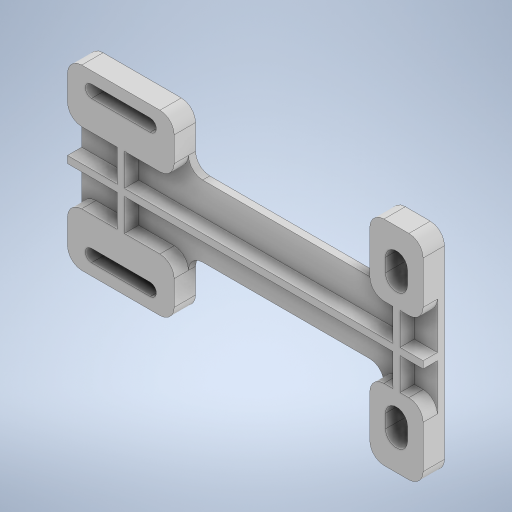
# Autodesk Inventor part: panel_holder
Saved by Autodesk Inventor 2023 (Build 270158000, 158)
## iProperties
Created: 2023-10-19
Part Number: panel_holder
Material: Generic
Document SubType Name: Modeling
Designer: mark
Density: 1 g/cm^3
Appearance: Default
Author: mark
Autodesk Inventor part; units mm, degrees
ref_plane "YZ Plane" through (0, 0, 0) normal (1, 0, 0) x (0, 1, 0)
ref_plane "XZ Plane" through (0, 0, 0) normal (0, 1, 0) x (-1, 0, 0)
ref_plane "XY Plane" through (0, 0, 0) normal (0, 0, 1) x (1, 0, 0)
sketch "Sketch1" plane through (0, 0, 0) normal (0, 0, 1) x (1, 0, 0)
  line L0 (0, 0) -> (-100, 0)
  line L1 (-100, 0) -> (-100, 50)
  line L2 (-100, 50) -> (0, 50)
  line L3 (0, 50) -> (0, 0)
  line L4 (-93.25, 46.75) -> (-76.75, 46.75)
  line L5 (-75, 45) -> (-75, 45)
  line L6 (-76.75, 43.25) -> (-93.25, 43.25)
  line L7 (-95, 45) -> (-95, 45)
  line L8 (-93.25, 6.75) -> (-76.75, 6.75)
  line L9 (-75, 5) -> (-75, 5)
  line L10 (-76.75, 3.25) -> (-93.25, 3.25)
  line L11 (-95, 5) -> (-95, 5)
  arc A0 (-93.25, 46.75) -> (-95, 45) centre (-93.25, 45) ccw
  arc A1 (-95, 45) -> (-93.25, 43.25) centre (-93.25, 45) ccw
  arc A2 (-75, 45) -> (-76.75, 46.75) centre (-76.75, 45) ccw
  arc A3 (-76.75, 43.25) -> (-75, 45) centre (-76.75, 45) ccw
  arc A4 (-75, 5) -> (-76.75, 6.75) centre (-76.75, 5) ccw
  arc A5 (-93.25, 6.75) -> (-95, 5) centre (-93.25, 5) ccw
  arc A6 (-95, 5) -> (-93.25, 3.25) centre (-93.25, 5) ccw
  arc A7 (-76.75, 3.25) -> (-75, 5) centre (-76.75, 5) ccw
  line L12 (0, 55) -> (-15, 55)
  line L13 (-15, 55) -> (-15, -5)
  line L14 (-15, -5) -> (0, -5)
  line L15 (0, -5) -> (0, 55)
  line L16 (-70, 50) -> (-15, 50)
  line L17 (-15, 50) -> (-15, 35)
  line L18 (-15, 35) -> (-70, 35)
  line L19 (-70, 35) -> (-70, 50)
  line L20 (-70, 0) -> (-15, 0)
  line L21 (-15, 0) -> (-15, 15)
  line L22 (-15, 15) -> (-70, 15)
  line L23 (-70, 15) -> (-70, 0)
  point P0 (-75, 43.25)
  point P1 (-75, 46.75)
  point P2 (-95, 43.25)
  point P3 (-95, 6.75)
  point P4 (-75, 3.25)
  point P5 (-75, 6.75)
  dimension "d0" = 100
  dimension "d1" = 50
  dimension "d2" = 20
  dimension "d3" = 3.5
  dimension "d4" = 3.5
  dimension "d5" = 36.5
  dimension "d6" = 3.25
  dimension "d7" = 5
  dimension "d8" = 1.75
  dimension "d11" = 15
  dimension "d12" = 60
  dimension "d13" = 15
  dimension "d14" = 15
  dimension "d17" = 55
  dimension "d18" = 15
  dimension "d19" = 5
  constraints: 48 end point, 19 point on line, 16 point on circle, 16 tangent, 12 parallel, 8 centre point, 7 equal radius, 6 horizontal, 6 perpendicular, 1 midpoint
  measures "d0" distance of L1.end L2.end
  measures "d1" distance of L0.end L1.end
  measures "d2" distance of point (-75, 43.25) point (-95, 43.25)
  measures "d3" distance of point (-75, 46.75) point (-75, 43.25)
  measures "d4" distance of point (-75, 6.75) point (-75, 3.25)
  measures "d5" distance between parallel lines of L8 L6
  measures "d6" distance between parallel lines of L0 L10
  measures "d7" distance from line of L1 point (-95, 5)
  measures "d8" radius of A0
  measures "d11" distance of L14.end L13.end
  measures "d12" distance of L12.end L13.end
  measures "d13" distance of L18.end L16.start
  measures "d14" distance of L22.end L20.start
  measures "d17" distance of L17.end L18.end
  measures "d18" distance between parallel lines of L3 L13
  measures "d19" distance between parallel lines of L2 L12
extrude "Extrusion1" add sketch "Sketch1" along normal blind 2 contours L15 L14 L13 L0 | L0 L13 L2 L3 | L2 L13 L12 L15 | L0 L1 L2 L19 L18 L13 L22 L23
fillet "Fillet1" radius 4 12 edges at (-70, 50, 1) (-70, 35, 1) (-100, 50, 1) (-100, 0, 1) (-70, 0, 1) (-70, 15, 1) (-15, 15, 1) (-15, 35, 1) (-15, 55, 1) (0, 55, 1) (0, -5, 1) (-15, -5, 1)
sketch "Sketch2" plane through (0, 0, 2) normal (0, 0, 1) x (1, 0, 0)
  line L0 (-7.5, 49) -> (-7.5, 49)
  line L1 (-4.4, 45.9) -> (-4.4, 42.1)
  line L2 (-7.5, 39) -> (-7.5, 39)
  line L3 (-10.6, 42.1) -> (-10.6, 45.9)
  line L4 (-7.5, 11) -> (-7.5, 11)
  line L5 (-4.4, 7.9) -> (-4.4, 4.1)
  line L6 (-7.5, 1) -> (-7.5, 1)
  line L7 (-10.6, 4.1) -> (-10.6, 7.9)
  line L8 (0, -1) -> (0, 51) projected
  line L9 (-4, 55) -> (-11, 55) projected
  line L10 (-11, -5) -> (-4, -5) projected
  arc A0 (-7.5, 49) -> (-10.6, 45.9) centre (-7.5, 45.9) ccw
  arc A1 (-4.4, 45.9) -> (-7.5, 49) centre (-7.5, 45.9) ccw
  arc A2 (-7.5, 39) -> (-4.4, 42.1) centre (-7.5, 42.1) ccw
  arc A3 (-10.6, 42.1) -> (-7.5, 39) centre (-7.5, 42.1) ccw
  arc A4 (-7.5, 11) -> (-10.6, 7.9) centre (-7.5, 7.9) ccw
  arc A5 (-7.5, 1) -> (-4.4, 4.1) centre (-7.5, 4.1) ccw
  arc A6 (-4.4, 7.9) -> (-7.5, 11) centre (-7.5, 7.9) ccw
  arc A7 (-10.6, 4.1) -> (-7.5, 1) centre (-7.5, 4.1) ccw
  point P0 (0, 0)
  point P1 (-4.4, 39)
  point P2 (-4.4, 49)
  point P3 (-10.6, 39)
  point P4 (-4.4, 1)
  point P5 (-4.4, 11)
  point P6 (-10.6, 1)
  point P7 (-7.5, 49)
  point P8 (-7.5, 1)
  point P9 (-7.5, 1)
  dimension "d21" = 6.2
  dimension "d22" = 10
  dimension "d23" = 6.2
  dimension "d24" = 10
  dimension "d25" = 4.4
  dimension "d26" = 4.4
  dimension "d27" = 6
  dimension "d28" = 6
  dimension "d29" = 3.1
  constraints: 16 end point, 16 point on circle, 16 tangent, 12 point on line, 8 centre point, 7 equal radius, 4 parallel, 2 horizontal, 2 midpoint, 2 perpendicular
  measures "d21" distance of point (-4.4, 39) point (-10.6, 39)
  measures "d22" distance of point (-4.4, 49) point (-4.4, 39)
  measures "d23" distance of point (-4.4, 1) point (-10.6, 1)
  measures "d24" distance of point (-4.4, 11) point (-4.4, 1)
  measures "d25" distance between parallel lines of L8 L1
  measures "d26" distance between parallel lines of L8 L5
  measures "d27" distance from line of L9 point (-7.5, 49)
  measures "d28" distance from line of L10 point (-7.5, 1)
  measures "d29" radius of A0
extrude "Extrusion2" cut sketch "Sketch2" against normal blind 2
sketch "Sketch3" plane through (0, 0, 2) normal (0, 0, 1) x (1, 0, 0)
  line L0 (0, -1) -> (0, 51) projected
  line L1 (-100, 24) -> (-100, 26)
  line L2 (0, 26) -> (0, 24)
  line L3 (-11, 55) -> (-4, 55)
  line L4 (0, 51) -> (0, 39)
  line L5 (-15, 39) -> (-15, 51)
  line L6 (-4, -5) -> (-11, -5)
  line L7 (-15, -1) -> (-15, 11)
  line L8 (0, 11) -> (0, -1)
  line L9 (-96, 50) -> (-74, 50)
  line L10 (-70, 46) -> (-70, 39)
  line L11 (-100, 39) -> (-100, 46)
  line L12 (-100, 46) -> (-100, 4) projected
  line L13 (-74, 0) -> (-96, 0)
  line L14 (-100, 4) -> (-100, 11)
  line L15 (-70, 11) -> (-70, 4)
  arc A0 (-96, 50) -> (-100, 46) centre (-96, 46) ccw
  arc A1 (-70, 46) -> (-74, 50) centre (-74, 46) ccw
  arc A2 (-100, 39) -> (-96, 35) centre (-96, 39) ccw
  arc A3 (-74, 35) -> (-70, 39) centre (-74, 39) ccw
  arc A4 (-96, 15) -> (-100, 11) centre (-96, 11) ccw
  arc A5 (-100, 4) -> (-96, 0) centre (-96, 4) ccw
  arc A6 (-74, 0) -> (-70, 4) centre (-74, 4) ccw
  arc A7 (-70, 11) -> (-74, 15) centre (-74, 11) ccw
  arc A8 (-11, 15) -> (-15, 11) centre (-11, 11) ccw
  arc A9 (0, 11) -> (-4, 15) centre (-4, 11) ccw
  arc A10 (-4, -5) -> (0, -1) centre (-4, -1) ccw
  arc A11 (-15, -1) -> (-11, -5) centre (-11, -1) ccw
  arc A12 (-15, 39) -> (-11, 35) centre (-11, 39) ccw
  arc A13 (-4, 35) -> (0, 39) centre (-4, 39) ccw
  arc A14 (0, 51) -> (-4, 55) centre (-4, 51) ccw
  arc A15 (-11, 55) -> (-15, 51) centre (-11, 51) ccw
  line L16 (-100, 26) -> (-86, 26)
  line L17 (-86, 35) -> (-86, 26)
  line L18 (-86, 24) -> (-86, 15)
  line L19 (-86, 24) -> (-100, 24)
  line L20 (-84, 15) -> (-84, 24)
  line L21 (-84, 26) -> (-84, 35)
  line L22 (-96, 15) -> (-86, 15)
  line L23 (-84, 15) -> (-74, 15)
  line L24 (-74, 35) -> (-84, 35)
  line L25 (-86, 35) -> (-96, 35)
  line L26 (-4, 35) -> (-6.5, 35)
  line L27 (-8.5, 35) -> (-11, 35)
  line L28 (-84, 26) -> (-8.5, 26)
  line L29 (-6.5, 26) -> (0, 26)
  line L30 (-8.5, 35) -> (-8.5, 26)
  line L31 (-8.5, 24) -> (-8.5, 15)
  line L32 (-6.5, 15) -> (-6.5, 24)
  line L33 (-6.5, 26) -> (-6.5, 35)
  line L34 (0, 24) -> (-6.5, 24)
  line L35 (-8.5, 24) -> (-84, 24)
  line L36 (-11, 15) -> (-8.5, 15)
  line L37 (-6.5, 15) -> (-4, 15)
  line L38 (-10.6, 45.9) -> (-10.6, 42.1) projected
  line L39 (-10.6, 45.9) -> (-10.6, 42.1)
  arc A16 (-10.6, 42.1) -> (-4.4, 42.1) centre (-7.5, 42.1) ccw projected
  arc A17 (-10.6, 42.1) -> (-4.4, 42.1) centre (-7.5, 42.1) ccw
  arc A18 (-4.4, 45.9) -> (-10.6, 45.9) centre (-7.5, 45.9) ccw projected
  arc A19 (-4.4, 45.9) -> (-10.6, 45.9) centre (-7.5, 45.9) ccw
  line L40 (-4.4, 45.9) -> (-4.4, 42.1)
  arc A20 (-4.4, 7.9) -> (-10.6, 7.9) centre (-7.5, 7.9) ccw projected
  arc A21 (-4.4, 7.9) -> (-10.6, 7.9) centre (-7.5, 7.9) ccw
  arc A22 (-10.6, 4.1) -> (-4.4, 4.1) centre (-7.5, 4.1) ccw projected
  arc A23 (-10.6, 4.1) -> (-4.4, 4.1) centre (-7.5, 4.1) ccw
  line L41 (-10.6, 7.9) -> (-10.6, 4.1) projected
  line L42 (-10.6, 7.9) -> (-10.6, 4.1)
  line L43 (-4.4, 4.1) -> (-4.4, 7.9) projected
  line L44 (-4.4, 4.1) -> (-4.4, 7.9)
  arc A24 (-93.25, 46.75) -> (-93.25, 43.25) centre (-93.25, 45) ccw projected
  line L45 (-93.25, 46.75) -> (-76.75, 46.75) projected
  line L46 (-93.25, 46.75) -> (-76.75, 46.75)
  arc A25 (-93.25, 46.75) -> (-93.25, 43.25) centre (-93.25, 45) ccw
  arc A26 (-76.75, 43.25) -> (-76.75, 46.75) centre (-76.75, 45) ccw
  line L47 (-76.75, 43.25) -> (-93.25, 43.25) projected
  line L48 (-93.25, 43.25) -> (-76.75, 43.25)
  arc A27 (-93.25, 6.75) -> (-93.25, 3.25) centre (-93.25, 5) ccw projected
  line L49 (-93.25, 6.75) -> (-76.75, 6.75)
  arc A28 (-76.75, 3.25) -> (-76.75, 6.75) centre (-76.75, 5) ccw projected
  arc A29 (-76.75, 3.25) -> (-76.75, 6.75) centre (-76.75, 5) ccw
  line L50 (-76.75, 3.25) -> (-93.25, 3.25)
  point P0 (0, 0)
  point P1 (0, 25)
  point P2 (0, 35)
  point P3 (0, 55)
  point P4 (0, -5)
  point P5 (-15, 15)
  point P6 (-15, -5)
  point P7 (-70, 35)
  point P8 (-100, 35)
  point P9 (-70, 0)
  point P10 (-100, 15)
  point P11 (-85, 35)
  point P12 (-7.5, 35)
  dimension "d32" = 100
  dimension "d33" = 2
  dimension "d35" = 20
  dimension "d36" = 20
  dimension "d37" = 4
  constraints: 88 end point, 46 point on circle, 46 tangent, 30 parallel, 23 centre point, 19 point on line, 15 equal radius, 9 horizontal, 7 perpendicular, 5 collinear, 1 midpoint
  measures "d32" distance of L1.end L2.start
  measures "d33" distance of L1.start L1.end
  measures "d35" distance of point (0, 55) point (0, 35)
  measures "d36" distance of point (-15, -5) point (-15, 15)
  measures "d37" radius of A0
extrude "Extrusion3" add sketch "Sketch3" along normal blind 4 contours A10 L6 A11 L7 A8 L36 L31 L35 L20 L23 A7 L15 A6 L13 A5 L12 A4 L22 L18 L19 L1 L16 L17 L25 A2 L11 A0 L9 A1 L10 A3 L24 L21 L28 L30 L27 A12 L5 A15 L3 A14 L0 A13 L26 L33 L29 L34 L32 L37 A9
equation "\"d26\" = d25"
equation "\"d34\" = 0.5 * d33"
equation "\"d38\" = d33"
equation "\"d39\" = 0.5 * d38"
equation "\"d40\" = d33"
equation "\"d41\" = 0.5 * d33"
body "Solid1"
